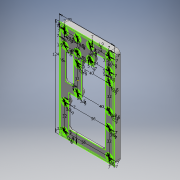
# Autodesk Inventor part: TxBoardMount
Saved by Autodesk Inventor 2016 (Build 200138000, 138)
## iProperties
Created: 2026-04-04
Part Number: TxBoardMount
Material: Generic
Document SubType Name: Modeling
Designer: Steve
Density: 1 g/cm^3
Appearance: Default
Author: Steve
Autodesk Inventor part; units mm, degrees
ref_plane "YZ Plane" through (0, 0, 0) normal (1, 0, 0) x (0, 1, 0)
ref_plane "XZ Plane" through (0, 0, 0) normal (0, 1, 0) x (-1, 0, 0)
ref_plane "XY Plane" through (0, 0, 0) normal (0, 0, 1) x (1, 0, 0)
sketch "Sketch1" plane through (0, 0, 0) normal (0, 1, 0) x (-1, 0, 0)
  line L0 (24.0391, 52.7087) -> (-45.9609, 52.7087)
  line L1 (-45.9609, 52.7087) -> (-45.9609, -71.2913)
  line L2 (-45.9609, -71.2913) -> (24.0391, -71.2913)
  line L3 (24.0391, -71.2913) -> (24.0391, 52.7087)
  line L4 (22.1391, 50.8087) -> (-44.0609, 50.8087)
  line L5 (-44.0609, 50.8087) -> (-44.0609, -69.3913)
  line L6 (-44.0609, -69.3913) -> (22.1391, -69.3913)
  line L7 (22.1391, -69.3913) -> (22.1391, 50.8087)
  circle A0 centre (17.0391, 45.7087) radius 4.5
  circle A1 centre (17.0391, 45.7087) radius 3.5
  circle A2 centre (17.0391, 45.7087) radius 1.75
  line L8 (18.7891, 42.6776) -> (15.2891, 42.6776)
  line L9 (15.2891, 42.6776) -> (13.5391, 45.7087)
  line L10 (13.5391, 45.7087) -> (15.2891, 48.7398)
  line L11 (15.2891, 48.7398) -> (18.7891, 48.7398)
  line L12 (18.7891, 48.7398) -> (20.5391, 45.7087)
  line L13 (20.5391, 45.7087) -> (18.7891, 42.6776)
  circle A3 centre (1.0391, 45.7087) radius 1.75
  circle A4 centre (1.0391, 45.7087) radius 3.5
  circle A5 centre (1.0391, 45.7087) radius 4.5
  circle A6 centre (-38.9609, 45.7087) radius 1.75
  circle A7 centre (-14.9609, 45.7087) radius 1.75
  circle A8 centre (-14.9609, 45.7087) radius 3.5
  circle A9 centre (-14.9609, 45.7087) radius 4.5
  circle A10 centre (-38.9609, 45.7087) radius 3.5
  circle A11 centre (-38.9609, 45.7087) radius 4.5
  line L14 (-0.7109, 42.6776) -> (-2.4609, 45.7087)
  line L15 (-2.4609, 45.7087) -> (-0.7109, 48.7398)
  line L16 (-0.7109, 48.7398) -> (2.7891, 48.7398)
  line L17 (2.7891, 48.7398) -> (4.5391, 45.7087)
  line L18 (4.5391, 45.7087) -> (2.7891, 42.6776)
  line L19 (2.7891, 42.6776) -> (-0.7109, 42.6776)
  line L20 (-16.7109, 42.6776) -> (-18.4609, 45.7087)
  line L21 (-18.4609, 45.7087) -> (-16.7109, 48.7398)
  line L22 (-16.7109, 48.7398) -> (-13.2109, 48.7398)
  line L23 (-13.2109, 48.7398) -> (-11.4609, 45.7087)
  line L24 (-11.4609, 45.7087) -> (-13.2109, 42.6776)
  line L25 (-13.2109, 42.6776) -> (-16.7109, 42.6776)
  line L26 (-40.7109, 42.6776) -> (-42.4609, 45.7087)
  line L27 (-42.4609, 45.7087) -> (-40.7109, 48.7398)
  line L28 (-40.7109, 48.7398) -> (-37.2109, 48.7398)
  line L29 (-37.2109, 48.7398) -> (-35.4609, 45.7087)
  line L30 (-35.4609, 45.7087) -> (-37.2109, 42.6776)
  line L31 (-37.2109, 42.6776) -> (-40.7109, 42.6776)
  circle A12 centre (-14.9609, 29.7087) radius 1.75
  circle A13 centre (1.0391, 29.7087) radius 1.75
  circle A14 centre (17.0391, 29.7087) radius 1.75
  circle A15 centre (-38.9609, 29.7087) radius 1.75
  circle A16 centre (17.0391, 29.7087) radius 3.5
  circle A17 centre (17.0391, 29.7087) radius 4.5
  circle A18 centre (1.0391, 29.7087) radius 3.5
  circle A19 centre (1.0391, 29.7087) radius 4.5
  circle A20 centre (-14.9609, 29.7087) radius 3.5
  circle A21 centre (-14.9609, 29.7087) radius 4.5
  circle A22 centre (-38.9609, 29.7087) radius 3.5
  circle A23 centre (-38.9609, 29.7087) radius 4.5
  line L32 (15.2891, 26.6776) -> (13.5391, 29.7087)
  line L33 (13.5391, 29.7087) -> (15.2891, 32.7398)
  line L34 (15.2891, 32.7398) -> (18.7891, 32.7398)
  line L35 (18.7891, 32.7398) -> (20.5391, 29.7087)
  line L36 (20.5391, 29.7087) -> (18.7891, 26.6776)
  line L37 (18.7891, 26.6776) -> (15.2891, 26.6776)
  line L38 (-0.7109, 26.6776) -> (-2.4609, 29.7087)
  line L39 (-2.4609, 29.7087) -> (-0.7109, 32.7398)
  line L40 (-0.7109, 32.7398) -> (2.7891, 32.7398)
  line L41 (2.7891, 32.7398) -> (4.5391, 29.7087)
  line L42 (4.5391, 29.7087) -> (2.7891, 26.6776)
  line L43 (2.7891, 26.6776) -> (-0.7109, 26.6776)
  line L44 (-16.7109, 26.6776) -> (-18.4609, 29.7087)
  line L45 (-18.4609, 29.7087) -> (-16.7109, 32.7398)
  line L46 (-16.7109, 32.7398) -> (-13.2109, 32.7398)
  line L47 (-13.2109, 32.7398) -> (-11.4609, 29.7087)
  line L48 (-11.4609, 29.7087) -> (-13.2109, 26.6776)
  line L49 (-13.2109, 26.6776) -> (-16.7109, 26.6776)
  line L50 (-40.7109, 26.6776) -> (-42.4609, 29.7087)
  line L51 (-42.4609, 29.7087) -> (-40.7109, 32.7398)
  line L52 (-40.7109, 32.7398) -> (-37.2109, 32.7398)
  line L53 (-37.2109, 32.7398) -> (-35.4609, 29.7087)
  line L54 (-35.4609, 29.7087) -> (-37.2109, 26.6776)
  line L55 (-37.2109, 26.6776) -> (-40.7109, 26.6776)
  circle A24 centre (-38.9609, 17.7087) radius 1.75
  circle A25 centre (1.0391, 17.7087) radius 1.75
  circle A26 centre (1.0391, -14.2913) radius 1.75
  circle A27 centre (-38.9609, -14.2913) radius 1.75
  circle A28 centre (1.0391, 17.7087) radius 3.5
  circle A29 centre (1.0391, 17.7087) radius 4.5
  circle A30 centre (1.0391, -14.2913) radius 3.5
  circle A31 centre (1.0391, -14.2913) radius 4.5
  circle A32 centre (-38.9609, 17.7087) radius 3.5
  circle A33 centre (-38.9609, 17.7087) radius 4.5
  circle A34 centre (-38.9609, -14.2913) radius 3.5
  circle A35 centre (-38.9609, -14.2913) radius 4.5
  line L56 (2.7891, 14.6776) -> (-0.7109, 14.6776)
  line L57 (-0.7109, 14.6776) -> (-2.4609, 17.7087)
  line L58 (-2.4609, 17.7087) -> (-0.7109, 20.7398)
  line L59 (-0.7109, 20.7398) -> (2.7891, 20.7398)
  line L60 (2.7891, 20.7398) -> (4.5391, 17.7087)
  line L61 (4.5391, 17.7087) -> (2.7891, 14.6776)
  line L62 (-0.7109, -17.3224) -> (-2.4609, -14.2913)
  line L63 (-2.4609, -14.2913) -> (-0.7109, -11.2602)
  line L64 (-0.7109, -11.2602) -> (2.7891, -11.2602)
  line L65 (2.7891, -11.2602) -> (4.5391, -14.2913)
  line L66 (4.5391, -14.2913) -> (2.7891, -17.3224)
  line L67 (2.7891, -17.3224) -> (-0.7109, -17.3224)
  line L68 (-40.7109, -17.3224) -> (-42.4609, -14.2913)
  line L69 (-42.4609, -14.2913) -> (-40.7109, -11.2602)
  line L70 (-40.7109, -11.2602) -> (-37.2109, -11.2602)
  line L71 (-37.2109, -11.2602) -> (-35.4609, -14.2913)
  line L72 (-35.4609, -14.2913) -> (-37.2109, -17.3224)
  line L73 (-37.2109, -17.3224) -> (-40.7109, -17.3224)
  line L74 (-40.7109, 14.6776) -> (-42.4609, 17.7087)
  line L75 (-42.4609, 17.7087) -> (-40.7109, 20.7398)
  line L76 (-40.7109, 20.7398) -> (-37.2109, 20.7398)
  line L77 (-37.2109, 20.7398) -> (-35.4609, 17.7087)
  line L78 (-35.4609, 17.7087) -> (-37.2109, 14.6776)
  line L79 (-37.2109, 14.6776) -> (-40.7109, 14.6776)
  circle A36 centre (-38.9609, -64.2913) radius 1.75
  circle A37 centre (-38.9609, -32.2913) radius 1.75
  circle A38 centre (17.0391, -64.2913) radius 1.75
  circle A39 centre (17.0391, -32.2913) radius 1.75
  circle A40 centre (17.0391, -32.2913) radius 3.5
  circle A41 centre (17.0391, -64.2913) radius 3.5
  circle A42 centre (-38.9609, -64.2913) radius 3.5
  circle A43 centre (-38.9609, -32.2913) radius 3.5
  circle A44 centre (17.0391, -32.2913) radius 4.5
  circle A45 centre (17.0391, -64.2913) radius 4.5
  circle A46 centre (-38.9609, -64.2913) radius 4.5
  circle A47 centre (-38.9609, -32.2913) radius 4.5
  line L80 (-40.7109, -35.3224) -> (-42.4609, -32.2913)
  line L81 (-42.4609, -32.2913) -> (-40.7109, -29.2602)
  line L82 (-40.7109, -29.2602) -> (-37.2109, -29.2602)
  line L83 (-37.2109, -29.2602) -> (-35.4609, -32.2913)
  line L84 (-35.4609, -32.2913) -> (-37.2109, -35.3224)
  line L85 (-37.2109, -35.3224) -> (-40.7109, -35.3224)
  line L86 (-40.7109, -67.3224) -> (-42.4609, -64.2913)
  line L87 (-42.4609, -64.2913) -> (-40.7109, -61.2602)
  line L88 (-40.7109, -61.2602) -> (-37.2109, -61.2602)
  line L89 (-37.2109, -61.2602) -> (-35.4609, -64.2913)
  line L90 (-35.4609, -64.2913) -> (-37.2109, -67.3224)
  line L91 (-37.2109, -67.3224) -> (-40.7109, -67.3224)
  line L92 (15.2891, -67.3224) -> (13.5391, -64.2913)
  line L93 (13.5391, -64.2913) -> (15.2891, -61.2602)
  line L94 (15.2891, -61.2602) -> (18.7891, -61.2602)
  line L95 (18.7891, -61.2602) -> (20.5391, -64.2913)
  line L96 (20.5391, -64.2913) -> (18.7891, -67.3224)
  line L97 (18.7891, -67.3224) -> (15.2891, -67.3224)
  line L98 (15.2891, -35.3224) -> (13.5391, -32.2913)
  line L99 (13.5391, -32.2913) -> (15.2891, -29.2602)
  line L100 (15.2891, -29.2602) -> (18.7891, -29.2602)
  line L101 (18.7891, -29.2602) -> (20.5391, -32.2913)
  line L102 (20.5391, -32.2913) -> (18.7891, -35.3224)
  line L103 (18.7891, -35.3224) -> (15.2891, -35.3224)
  line L104 (-19.9609, 40.7087) -> (-33.9609, 40.7087)
  line L105 (-33.9609, 40.7087) -> (-33.9609, -59.2913)
  line L106 (-33.9609, -59.2913) -> (12.0391, -59.2913)
  line L107 (12.0391, -59.2913) -> (12.0391, -19.2913)
  line L108 (12.0391, -19.2913) -> (-3.9609, -19.2913)
  line L109 (-3.9609, -19.2913) -> (-3.9609, 24.7087)
  line L110 (-3.9609, 24.7087) -> (-19.9609, 24.7087)
  line L111 (-19.9609, 24.7087) -> (-19.9609, 40.7087)
  line L112 (16.1391, 24.7087) -> (6.0391, 24.7087)
  line L113 (6.0391, 24.7087) -> (6.0391, -9.2913)
  line L114 (6.0391, -9.2913) -> (16.1391, -9.2913)
  line L115 (16.1391, -9.2913) -> (16.1391, 24.7087)
  point P0 (0, 0)
  dimension "d7" = 7
  dimension "d12" = 7
  dimension "d22" = 7
  dimension "d24" = 7
  dimension "d38" = 7
  dimension "d40" = 7
  dimension "d42" = 7
  dimension "d44" = 7
  dimension "d58" = 7
  dimension "d60" = 7
  dimension "d62" = 7
  dimension "d64" = 7
  dimension "d78" = 7
  dimension "d79" = 7
  dimension "d80" = 7
  dimension "d81" = 7
  dimension "d0" = 1.9
  dimension "d1" = 1.9
  dimension "d2" = 1.9
  dimension "d3" = 1.9
  dimension "d4" = 124
  dimension "d5" = 70
  dimension "d6" = 9
  dimension "d8" = 3.5
  dimension "d9" = 7
  dimension "d10" = 7
  dimension "d11" = 3.5
  dimension "d13" = 9
  dimension "d14" = 7
  dimension "d15" = 3.5
  dimension "d16" = 7
  dimension "d17" = 7
  dimension "d18" = 3.5
  dimension "d19" = 7
  dimension "d20" = 16
  dimension "d21" = 24
  dimension "d23" = 9
  dimension "d25" = 9
  dimension "d26" = 3.5
  dimension "d27" = 3.5
  dimension "d28" = 3.5
  dimension "d29" = 3.5
  dimension "d30" = 7
  dimension "d31" = 16
  dimension "d32" = 16
  dimension "d33" = 16
  dimension "d34" = 16
  dimension "d35" = 7
  dimension "d36" = 24
  dimension "d37" = 16
  dimension "d39" = 9
  dimension "d41" = 9
  dimension "d43" = 9
  dimension "d45" = 9
  dimension "d46" = 3.5
  dimension "d47" = 3.5
  dimension "d48" = 3.5
  dimension "d49" = 3.5
  dimension "d50" = 7
  dimension "d51" = 7
  dimension "d52" = 12
  dimension "d53" = 12
  dimension "d54" = 40
  dimension "d55" = 32
  dimension "d56" = 32
  dimension "d57" = 40
  dimension "d59" = 9
  dimension "d61" = 9
  dimension "d63" = 9
  dimension "d65" = 9
  dimension "d66" = 3.5
  dimension "d67" = 3.5
  dimension "d68" = 7
  dimension "d69" = 7
  dimension "d70" = 7
  dimension "d71" = 32
  dimension "d72" = 3.5
  dimension "d73" = 3.5
  dimension "d74" = 7
  dimension "d75" = 32
  constraints: 232 end point, 48 coincident, 32 centre point, 11 perpendicular, 9 point on line, 5 horizontal, 4 parallel, 256 other
  measures "d0" distance between parallel lines of L3 L7
  measures "d1" distance between parallel lines of L6 L2
  measures "d2" distance between parallel lines of L5 L1
  measures "d3" distance between parallel lines of L0 L4
  measures "d4" distance of L2.end L0.start
  measures "d5" distance of L0.start L0.end
  measures "d6" diameter of A0
  measures "d8" diameter of A2
  measures "d9" distance from line of L3 A0.centre
  measures "d10" distance from line of L0 A0.centre
  measures "d11" diameter of A3
  measures "d13" diameter of A5
  measures "d14" distance from line of L0 A3.centre
  measures "d15" diameter of A6
  measures "d16" distance from line of L1 A6.centre
  measures "d17" distance from line of L0 A6.centre
  measures "d18" diameter of A7
  measures "d19" distance from line of L0 A7.centre
  measures "d20" distance of A3.centre A0.centre
  measures "d21" distance of A7.centre A6.centre
  measures "d23" diameter of A9
  measures "d25" diameter of A11
  measures "d26" diameter of A15
  measures "d27" diameter of A12
  measures "d28" diameter of A13
  measures "d29" diameter of A14
  measures "d30" distance from line of L3 A14.centre
  measures "d31" distance of A14.centre A0.centre
  measures "d32" distance of A13.centre A3.centre
  measures "d33" distance of A12.centre point (-14.961, 45.709)
  measures "d34" distance of A15.centre A6.centre
  measures "d35" distance from line of L1 A15.centre
  measures "d36" distance of A12.centre A15.centre
  measures "d37" distance of A13.centre A14.centre
  measures "d39" diameter of A17
  measures "d41" diameter of A19
  measures "d43" diameter of A21
  measures "d45" diameter of A23
  measures "d46" diameter of A24
  measures "d47" diameter of A25
  measures "d48" diameter of A26
  measures "d49" diameter of A27
  measures "d50" distance from line of L1 A24.centre
  measures "d51" distance from line of L1 A27.centre
  measures "d52" distance of A24.centre A15.centre
  measures "d53" distance of A25.centre point (1.039, 29.709)
  measures "d54" distance of A25.centre A24.centre
  measures "d55" distance of A27.centre A24.centre
  measures "d56" distance of A26.centre A25.centre
  measures "d57" distance of A27.centre A26.centre
  measures "d59" diameter of A29
  measures "d61" diameter of A31
  measures "d63" diameter of A33
  measures "d65" diameter of A35
  measures "d66" diameter of A36
  measures "d67" diameter of A37
  measures "d68" distance from line of L1 A36.centre
  measures "d69" distance from line of L2 A36.centre
  measures "d70" distance from line of L1 A37.centre
  measures "d71" distance of A37.centre A36.centre
  measures "d72" diameter of A39
  measures "d73" diameter of A38
  measures "d74" distance from line of L2 A38.centre
  measures "d75" distance of A38.centre A39.centre
extrude "Extrusion3" add sketch "Sketch1" along normal blind 7.5 contours L3 L2 L1 L0
extrude "Extrusion4" add sketch "Sketch1" along normal blind 2 contours L7 L6 L5 L4
extrude "Extrusion5" add sketch "Sketch1" along normal blind 4 contours A0 | A5 | A9 | A11 | A17 | A19 | A21 | A23 | A29 | A31 | A33 | A35 | A44 | A45 | A46 | A47
extrude "Extrusion6" add sketch "Sketch1" along normal blind 6 contours L12 A1 | L13 L8 L9 L10 L11 L12 | A1 L13 | L11 A1 | A1 L8 | L10 A1 | A1 L9 | L17 A4 | L18 L19 L14 L15 L16 L17 | A4 L18 | L16 A4 | A4 L19 | L15 A4 | A4 L14 | L23 A8 | L24 L25 L20 L21 L22 L23 | A8 L24 | L22 A8 | A8 L25 | L21 A8 | A8 L20 | L29 A10 | L30 L31 L26 L27 L28 L29 | A10 L30 | L28 A10 | A10 L31 | L27 A10 | A10 L26 | L35 A16 | L36 L37 L32 L33 L34 L35 | A16 L36 | L34 A16 | A16 L37 | L33 A16 | A16 L32 | L41 A18 | L42 L43 L38 L39 L40 L41 | A18 L42 | L40 A18 | A18 L43 | L39 A18 | A18 L38 | L47 A20 | L48 L49 L44 L45 L46 L47 | A20 L48 | L46 A20 | A20 L49 | L45 A20 | A20 L44 | L53 A22 | L54 L55 L50 L51 L52 L53 | A22 L54 | L52 A22 | A22 L55 | L51 A22 | A22 L50 | L60 A28 | L61 L56 L57 L58 L59 L60 | A28 L61 | L59 A28 | A28 L56 | L58 A28 | A28 L57 | L65 A30 | L66 L67 L62 L63 L64 L65 | A30 L66 | L64 A30 | A30 L67 | L63 A30 | A30 L62 | L77 A32 | L78 L79 L74 L75 L76 L77 | A32 L78 | L76 A32 | A32 L79 | L75 A32 | A32 L74 | L71 A34 | L72 L73 L68 L69 L70 L71 | A34 L72 | L70 A34 | A34 L73 | L69 A34 | A34 L68 | L101 A40 | L102 L103 L98 L99 L100 L101 | A40 L102 | L100 A40 | A40 L103 | L99 A40 | A40 L98 | L95 A41 | L96 L97 L92 L93 L94 L95 | A41 L96 | L94 A41 | A41 L97 | L93 A41 | A41 L92 | L89 A42 | L90 L91 L86 L87 L88 L89 | A42 L90 | L88 A42 | A42 L91 | L87 A42 | A42 L86 | L83 A43 | L84 L85 L80 L81 L82 L83 | A43 L84 | L82 A43 | A43 L85 | L81 A43 | A43 L80
extrude "Extrusion7" cut sketch "Sketch1" along normal blind 3 contours L13 L8 L9 L10 L11 L12 | L18 L19 L14 L15 L16 L17 | L24 L25 L20 L21 L22 L23 | L30 L31 L26 L27 L28 L29 | L36 L37 L32 L33 L34 L35 | L42 L43 L38 L39 L40 L41 | L48 L49 L44 L45 L46 L47 | L54 L55 L50 L51 L52 L53 | L61 L56 L57 L58 L59 L60 | L66 L67 L62 L63 L64 L65 | L78 L79 L74 L75 L76 L77 | L72 L73 L68 L69 L70 L71 | L102 L103 L98 L99 L100 L101 | L96 L97 L92 L93 L94 L95 | L90 L91 L86 L87 L88 L89 | L84 L85 L80 L81 L82 L83
fillet "Fillet1" radius 5 8 edges at (-22.1391, 4.75, 50.8087) (-22.1391, 4.75, -69.3913) (44.0609, 4.75, -69.3913) (44.0609, 4.75, 50.8087) (-24.0391, 3.75, -71.2913) (-24.0391, 3.75, 52.7087) (45.9609, 3.75, 52.7087) (45.9609, 3.75, -71.2913)
fillet "Fillet2" radius 3 12 edges at (33.9609, 1, -59.2913) (-12.0391, 1, -59.2913) (-12.0391, 1, -19.2913) (3.9609, 1, -19.2913) (19.9609, 1, 24.7087) (3.9609, 1, 24.7087) (-6.0391, 1, -9.2913) (-16.1391, 1, -9.2913) (-16.1391, 1, 24.7087) (-6.0391, 1, 24.7087) (33.9609, 1, 40.7087) (19.9609, 1, 40.7087)
body "Solid2"
